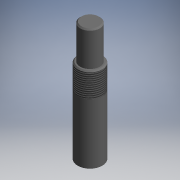
# Autodesk Inventor part: ESBF-BS-40-ESBF-BS-40---(KSA)
Saved by Autodesk Inventor 2017.3 (Build 213256000, 256)
## iProperties
Part Number: ESBF-BS-40-ESBF-BS-40---(KSA)
Material: Generic
Catalog Web Link: www.cadenas.de
Description: ESBF-(KSA)-Electro-cylinder
Vendor: FESTO
Document SubType Name: Modeling
Designer: partserver
Manufacturer: FESTO
Mass: 3.39925 g
Surface Area: 15.7322 cm^2
Volume: 3.39925 cm^3
Density: 1 g/cm^3
Appearance: PSOLRGB-128-128-128
Category: PARTsolutions
Company: FESTO
Title: ESBF-BS-40-ESBF-BS-40---(KSA)
Author: Cadenas PARTsolutions
Comments: Electro-cylinder
PSOL_IDENT_0: {$CADENAS_DATA\23d-libs\festo\parts\e\esbf\parts\esbf_ksa.prj},202 {VTYP=3D},{NB=ESBF-BS-40-ESBF-BS-
PSOL_IDENT_1: 40---(KSA)},{LINA=ESBF-BS-40-ESBF-BS-40---(KSA)},{NN=ESBF-(KSA)},{DATE=13.05.2020 13:32:49},{GEOMDAT
PSOL_IDENT_2: E=02.09.2015 14:29:35},{VERSION=},{LINEID=50},{WBVAR=},{WBNUMERIC=}  {NB=ESBF-BS-40-ESBF-BS-40---(KS
PSOL_IDENT_3: A)},{LINA=ESBF-BS-40-ESBF-BS-40---(KSA)},{KT=DUMMY},{TNR=8022585},{TYP=ESBF-BS-40},{KDM=40},{D2=8.00
PSOL_IDENT_4: 0},{L3=18.400},{L4=14.000},{G=30.000},{G1=30.000},{GUA=10.000},{P=0.750}
NB: ESBF-BS-40-ESBF-BS-40---(KSA)
NN: ESBF-(KSA)
NT: Electro-cylinder
NBSYN: $TYP.-$TYP.---(KSA)
LINA: ESBF-BS-40-ESBF-BS-40---(KSA)
CATALOG: Festo
TNR: 8022585
TYP: ESBF-BS-40
KDM: 40
D2: 8
L3: 18.4
L4: 14
G: 30
G1: 30
GUA: 10
P: 0.75
SUPPLIER: FESTO
ARTICLENO: ESBF-BS-40-ESBF-BS-40---(KSA)
BOMINFO: ESBF-BS-40-ESBF-BS-40---(KSA)
CREATOR: CADENAS GmbH
Autodesk Inventor part; units mm, degrees
sketch "Sketch_1" plane through (0, 0, 0) normal (1, 0, 0) x (0, 1, 0)
  line L0 (0, -48.4) -> (0, 0)
  line L1 (0, 0) -> (5, 0)
  line L2 (5, 0) -> (5, -33.94)
  line L3 (5, -33.94) -> (4.54, -34.4)
  line L4 (4.54, -34.4) -> (4, -34.4)
  line L5 (4, -34.4) -> (4, -47.9)
  line L6 (4, -47.9) -> (3.5, -48.4)
  line L7 (3.5, -48.4) -> (0, -48.4)
  line L8 (0, -48.4) -> (0, 0)
  constraints: 18 end point
revolve "Revolution1" add sketch "Sketch_1" angle 360 about axis through (0, 0, -48.4) along (0, 0, -1)
thread "Thread1" size "M10x0.75" class "6g" standard "ISO Metric profile" length 9.54
ref_plane "ANBAU_XY" through (0, 0, 0) normal (0, 0, 1) x (1, 0, 0)
ref_plane "ANBAU_YZ" through (0, 0, 0) normal (1, 0, 0) x (0, 1, 0)
ref_plane "ANBAU_ZX" through (0, 0, 0) normal (0, 1, 0) x (0, 0, 1)
body "Solid1"
